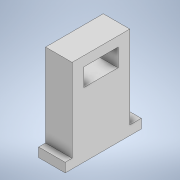
# Autodesk Inventor part: SecondaryBracket
Saved by Autodesk Inventor 2021 (Build 250183000, 183)
## iProperties
Created: 2022-01-19
Part Number: SecondaryBracket
Material: Generic
Document SubType Name: Modeling
Designer: Tlar613
Density: 1 g/cm^3
Appearance: Default
Author: Tlar613
Autodesk Inventor part; units mm, degrees
ref_plane "YZ Plane" through (0, 0, 0) normal (1, 0, 0) x (0, 1, 0)
ref_plane "XZ Plane" through (0, 0, 0) normal (0, 1, 0) x (-1, 0, 0)
ref_plane "XY Plane" through (0, 0, 0) normal (0, 0, 1) x (1, 0, 0)
sketch "Sketch1" plane through (0, 0, 0) normal (1, 0, 0) x (0, 1, 0)
  line L0 (0, 0) -> (40, 0)
  line L1 (40, 0) -> (40, 25)
  line L2 (40, 25) -> (0, 25)
  line L3 (0, 25) -> (0, 0)
  line L4 (35.8, 19.9) -> (28, 19.9)
  line L5 (28, 19.9) -> (28, 5.1)
  line L6 (28, 5.1) -> (35.8, 5.1)
  line L7 (35.8, 5.1) -> (35.8, 19.9)
  dimension "d0" = 40
  dimension "d1" = 25
  dimension "d2" = 14.8
  dimension "d3" = 7.8
  dimension "d4" = 5.1
  dimension "d5" = 28
  constraints: 16 end point, 4 parallel, 2 horizontal, 2 perpendicular
  measures "d0" distance of L1.end L2.end
  measures "d1" distance of L0.end L1.end
  measures "d2" distance of L6.end L4.start
  measures "d3" distance of L4.start L4.end
  measures "d4" distance between parallel lines of L2 L4
  measures "d5" distance between parallel lines of L3 L5
extrude "Extrusion1" add sketch "Sketch1" along normal blind 11.5
sketch "Sketch2" plane through (0, 0, 25) normal (0, 0, 1) x (1, 0, 0)
  line L0 (0, 0) -> (11.5, 0) projected
  line L1 (11.5, 40) -> (11.5, 0) projected
  line L2 (0, 0) -> (11.5, 0)
  line L3 (11.5, 0) -> (11.5, 4)
  line L4 (11.5, 4) -> (0, 4)
  line L5 (0, 4) -> (0, 0)
  dimension "d8" = 4
  constraints: 8 end point, 2 parallel, 1 horizontal, 1 perpendicular, 1 point on line
  measures "d8" distance between parallel lines of L0 L4
extrude "Extrusion2" add sketch "Sketch2" along normal blind 3
sketch "Sketch3" plane through (0, 0, 0) normal (0, 0, -1) x (-1, 0, 0)
  line L0 (0, 4) -> (-11.5, 4) projected
  line L1 (0, 4) -> (0, 0) projected
  line L2 (-11.5, 4) -> (0, 4)
  line L3 (0, 4) -> (0, 0)
  line L4 (0, 0) -> (-11.5, 0)
  line L5 (-11.5, 0) -> (-11.5, 4)
  constraints: 8 end point, 2 parallel, 1 horizontal, 1 perpendicular
extrude "Extrusion3" add sketch "Sketch3" along normal blind 5
body "Solid1"
